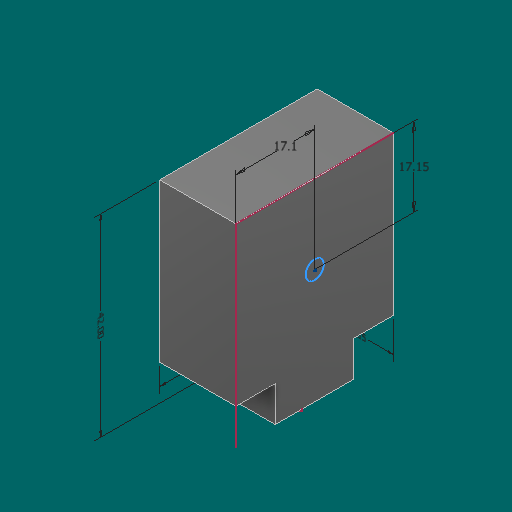
# Autodesk Inventor part: Arducam_Mega
Saved by Autodesk Inventor 2025.2 (Build 292293000, 293)
## iProperties
Created: 2025-04-19
Part Number: Arducam_Mega
Material: Generic
Document SubType Name: Modeling
Designer: Matt Caldwell
Density: 1 g/cm^3
Appearance: Default
Author: Matt Caldwell
Autodesk Inventor part; units mm, degrees
ref_plane "YZ Plane" through (0, 0, 0) normal (1, 0, 0) x (0, 1, 0)
ref_plane "XZ Plane" through (0, 0, 0) normal (0, 1, 0) x (-1, 0, 0)
ref_plane "XY Plane" through (0, 0, 0) normal (0, 0, 1) x (1, 0, 0)
sketch "Sketch1" plane through (0, 0, 0) normal (0, 1, 0) x (-1, 0, 0)
  line L0 (4.3357, 14.1429) -> (-12.2143, 14.1429)
  line L1 (-12.2143, 14.1429) -> (-12.2143, -20.0571)
  line L2 (-12.2143, -20.0571) -> (4.3357, -20.0571)
  line L3 (4.3357, -20.0571) -> (4.3357, 14.1429)
  point P0 (0, 0)
  dimension "d0" = 34.2
  dimension "d1" = 16.55
  constraints: 8 end point, 2 parallel, 1 horizontal, 1 perpendicular
  measures "d0" distance between parallel lines of L2 L0
  measures "d1" distance between parallel lines of L1 L3
extrude "Extrusion1" add sketch "Sketch1" along normal blind 42
sketch "Sketch2" plane through (12.2143, 0, 14.1429) normal (1, 0, 0) x (0, 0, -1)
  circle A0 centre (17.1, 24.85) radius 1.9655
  line L0 (0, 42) -> (34.2, 42) projected
  line L1 (0, 0) -> (0, 42) projected
  point P0 (14.1429, 0)
  dimension "d4" = 17.15
  dimension "d5" = 17.1
  constraints: 1 centre point
  measures "d4" distance from line of L0 A0.centre
  measures "d5" distance from line of L1 A0.centre
sketch "Sketch3" plane through (12.2143, 0, 14.1429) normal (1, 0, 0) x (0, 0, -1)
  line L0 (0, 0) -> (8.53, 0)
  line L1 (8.53, 0) -> (8.53, 7.7)
  line L2 (8.53, 7.7) -> (0, 7.7)
  line L3 (0, 7.7) -> (0, 0)
  point P0 (14.1429, 0)
  dimension "d18" = 7.7
  dimension "d19" = 8.53
  constraints: 8 end point, 2 parallel, 1 horizontal, 1 perpendicular
  measures "d18" distance between parallel lines of L0 L2
  measures "d19" distance between parallel lines of L3 L1
extrude "Extrusion2" cut sketch "Sketch3" against normal blind 17.9375
sketch "Sketch4" plane through (12.2143, 0, -20.0571) normal (1, 0, 0) x (0, 0, -1)
  line L0 (0, 0) -> (0, 42) projected
  line L1 (0, 0) -> (-8.6, 0)
  line L2 (-8.6, 0) -> (-8.6, 7.7)
  line L3 (-8.6, 7.7) -> (0, 7.7)
  line L4 (0, 7.7) -> (0, 0)
  point P0 (-20.0571, 0)
  point P1 (0, 7.7)
  dimension "d22" = 8.6
  dimension "d23" = 7.7
  constraints: 8 end point, 2 parallel, 1 horizontal, 1 perpendicular
  measures "d22" distance between parallel lines of L0 L2
  measures "d23" distance between parallel lines of L1 L3
extrude "Extrusion3" cut sketch "Sketch4" against normal blind 17.9375
body "Solid1"
